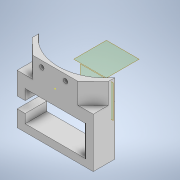
# Autodesk Inventor part: brazo_articulado_2
Saved by Autodesk Inventor 2021 (Build 250183000, 183)
## iProperties
Created: 2021-04-15
Part Number: brazo_articulado_2
Material: Genérico
Document SubType Name: Modeling
Designer: Joaquín
Density: 1 g/cm^3
Appearance: Valor por defecto
Author: Joaquín
Autodesk Inventor part; units mm, degrees
ref_plane "YZ Plane" through (0, 0, 0) normal (1, 0, 0) x (0, 1, 0)
ref_plane "XZ Plane" through (0, 0, 0) normal (0, 1, 0) x (-1, 0, 0)
ref_plane "XY Plane" through (0, 0, 0) normal (0, 0, 1) x (1, 0, 0)
ref_plane "Plano de trabajo1" through (16, 0, 22.5) normal (0, 0, -1) x (-1, 0, 0)
sketch "Boceto2" plane through (16, 0, 22.5) normal (0, 0, -1) x (-1, 0, 0)
  line L0 (-6.5, 0) -> (0, 0) projected
  line L1 (0, 0) -> (32, 0) projected
  circle A0 centre (8, 8) radius 1.5
  circle A1 centre (24, 8) radius 1.5
  point P0 (16, 0)
  dimension "d15" = 3
  dimension "d16" = 3
  constraints: 2 centre point
  measures "d15" diameter of A0
  measures "d16" diameter of A1
extrude "Extrusión2" [suppressed]
ref_plane "Plano de trabajo2" through (0, 0, 0) normal (0, -1, 0) x (1, 0, 0)
sketch "Boceto4" plane through (0, 0, 0) normal (0, -1, 0) x (1, 0, 0)
  circle A0 centre (0, 0) radius 32.5
  arc A1 (28.2887, 16) -> (-28.2887, 16) centre (0, 0) ccw projected
  line L0 (0, 32.5) -> (0, 34.5)
  line L1 (0, 34.5) -> (-26.2329, 34.5)
  line L2 (-26.2329, 34.5) -> (30.7149, 34.5)
  line L3 (0, 0) -> (0, 20)
  arc A2 (28.2887, 16) -> (-28.2887, 16) centre (0, 0) ccw projected
  line L4 (0, 20) -> (50, 20)
  line L5 (50, 20) -> (-50, 20)
  line L6 (0, 34.5) -> (15, 34.5)
  line L7 (15, 34.5) -> (25.6174, 20)
  line L8 (0, 34.5) -> (-15, 34.5)
  line L9 (-15, 34.5) -> (-25.6174, 20)
  point P0 (-25.6174, 20)
  dimension "d19" = 2
  dimension "d20" = 20
  dimension "d21" = 50
  dimension "d22" = 100
  dimension "d23" = 15
  dimension "d24" = 15
  constraints: 20 end point, 6 point on line, 3 point on circle, 2 vertical, 1 centre point, 1 coincident, 1 horizontal, 1 perpendicular
  measures "d19" distance of L0.start L0.end
  measures "d20" distance of L3.start L3.end
  measures "d21" distance of L3.end L4.end
  measures "d22" distance of L4.end L5.end
  measures "d23" distance of L0.end L6.end
  measures "d24" distance of L0.end L8.end
extrude "Extrusión3" add sketch "Boceto4" against normal blind 12 contours A0 L0 L2 L7 | L9 L1 L0 A0
sketch "Boceto5" plane through (-15, 0, 34.5) normal (0, 0, 1) x (1, 0, 0)
  line L0 (30, 0) -> (30, 12) projected
  line L1 (30, 0) -> (30, 8)
  line L2 (30, 8) -> (22, 8)
  line L3 (22, 8) -> (6, 8)
  circle A0 centre (22, 8) radius 1.5
  circle A1 centre (6, 8) radius 1.5
  point P0 (15, 0)
  dimension "d27" = 8
  dimension "d28" = 8
  dimension "d29" = 16
  dimension "d30" = 3
  dimension "d31" = 3
  constraints: 6 end point, 2 centre point, 2 coincident, 2 point on line, 1 perpendicular
  measures "d27" distance of L0.start L1.end
  measures "d28" distance of L1.end L2.end
  measures "d29" distance of L2.end L3.end
  measures "d30" diameter of A0
  measures "d31" diameter of A1
extrude "Extrusión4" cut sketch "Boceto5" against normal blind 12
sketch "Boceto6" plane through (0, 0, 0) normal (0, -1, 0) x (1, 0, 0)
  circle A0 centre (0, 0) radius 32.5
  arc A1 (25.6174, 20) -> (-25.6174, 20) centre (0, 0) ccw projected
  line L0 (-15, 34.5) -> (15, 34.5) projected
  line L1 (25.6174, 20) -> (15, 34.5)
  line L2 (15, 34.5) -> (-15, 34.5)
  line L3 (-15, 34.5) -> (-25.6174, 20)
  constraints: 6 end point, 1 centre point, 1 coincident, 1 collinear, 1 point on circle
extrude "Extrusión5" add sketch "Boceto6" along normal blind 2 contours A0 L3 L0 L1
sketch "Boceto7" plane through (0, -2, 0) normal (0, -1, 0) x (1, 0, 0)
  line L0 (-25.6174, 20) -> (-15, 34.5) projected
  line L1 (-15, 34.5) -> (-25.6174, 34.5)
  line L2 (-25.6174, 34.5) -> (-25.6174, 20)
  line L3 (-25.6174, 20) -> (25.6174, 20)
  line L4 (25.6174, 20) -> (25.6174, 34.5)
  line L5 (25.6174, 20) -> (15, 34.5) projected
  line L6 (15, 34.5) -> (25.6174, 34.5)
  circle A0 centre (0, 0) radius 32.5
  line L7 (-15, 34.5) -> (15, 34.5)
  constraints: 12 end point, 3 horizontal, 3 perpendicular, 1 coincident, 1 point on line, 3 other
extrude "Extrusión6" add sketch "Boceto7" along normal blind 8 contours L2 L1 L0 | A0 L3 | L0 L7 L5 A0 | L5 L6 L4 picked at (-1.7193, 25.9173)
sketch "Boceto8" plane through (-15, 12, 34.5) normal (0, 0, 1) x (1, 0, 0)
  line L0 (40.6174, -22) -> (-10.6174, -22) projected
  line L1 (-10.6174, -22) -> (-10.6174, -42.5)
  line L2 (-10.6174, -42.5) -> (39.7361, -42.5)
  line L3 (40.6174, -22) -> (40.6174, -42.5)
  line L4 (40.6174, -42.5) -> (39.7361, -42.5)
  line L5 (-10.6174, -22) -> (40.6174, -22) projected
  line L6 (40.6174, -14) -> (40.6174, -22) projected
  line L7 (-10.6174, -22) -> (40.6174, -22)
  line L8 (15, -22) -> (35.2, -22)
  line L9 (35.2, -22) -> (35.2, -42.5)
  line L10 (15, -22) -> (-5.2, -22)
  line L11 (-5.2, -22) -> (-5.2, -42.5)
  line L12 (-5.2, -42.5) -> (-5.2, -37.5)
  line L13 (-5.2, -22) -> (-5.2, -29)
  line L14 (-5.2, -29) -> (-10.6174, -29)
  line L15 (-5.2, -42.5) -> (-5.2, -36.5)
  line L16 (-5.2, -36.5) -> (-10.6174, -36.5)
  point P0 (15, -12)
  dimension "d38" = 20.5
  dimension "d39" = 20.5
  dimension "d40" = 20.2
  dimension "d41" = 20.2
  dimension "d43" = 7
  dimension "d44" = 6
  constraints: 28 end point, 9 point on line, 5 perpendicular, 2 vertical, 1 horizontal, 1 midpoint
  measures "d38" distance of L0.end L1.end
  measures "d39" distance of L0.start L3.end
  measures "d40" distance of L8.start L8.end
  measures "d41" distance of L8.start L10.end
  measures "d43" distance of L10.end L13.end
  measures "d44" distance of L11.end L15.end
extrude "Extrusión7" add sketch "Boceto8" against normal blind 14.5 contours L3 L4 L2 L9 L0 | L11 L14 L1 L0 | L2 L1 L16 L11
sketch "Boceto9" plane through (20.2, -30.5, 34.5) normal (0, -1, 0) x (1, 0, 0)
  line L0 (5.4174, -14.5) -> (5.4174, 0) projected
  line L1 (-45.8174, 0) -> (-45.8174, -14.5) projected
  line L2 (5.4174, 0) -> (-45.8174, 0)
  line L3 (-45.8174, 0) -> (-45.8174, -14.5)
  line L4 (-45.8174, -14.5) -> (5.4174, -14.5)
  line L5 (5.4174, 0) -> (-5.2, 0) projected
  line L6 (5.4174, -14.5) -> (5.4174, 0)
  point P0 (-20.2, -34.5)
  constraints: 8 end point, 2 perpendicular, 1 collinear, 1 horizontal
extrude "Extrusión8" add sketch "Boceto9" along normal blind 5
sketch "Boceto10" plane through (0, -2, 0) normal (0, 1, 0) x (1, 0, 0)
  line L0 (-15, -34.5) -> (-25.6174, -34.5) projected
  line L1 (-15, -34.5) -> (-25.6174, -34.5)
  line L2 (-25.6174, -34.5) -> (-25.6174, -24.5)
  line L3 (-25.6174, -34.5) -> (-25.6174, -20) projected
  line L4 (-25.6174, -24.5) -> (-15, -34.5)
  line L5 (-25.6174, -20) -> (25.6174, -20) projected
  line L6 (-25.6174, -24.5) -> (-25.6174, -20)
  line L7 (-25.6174, -20) -> (-15, -34.5)
  line L8 (-15, -34.5) -> (-25.6174, -20) projected
  arc A0 (-25.6174, -20) -> (25.6174, -20) centre (0, 0) ccw projected
  line L9 (0, -32.5) -> (0, -25.3096)
  line L10 (15, -34.5) -> (25.6174, -34.5)
  line L11 (25.6174, -34.5) -> (25.6174, -24.5)
  line L12 (25.6174, -34.5) -> (25.6174, -20)
  line L13 (25.6174, -24.5) -> (15, -34.5)
  line L14 (25.6174, -20) -> (15, -34.5)
  dimension "d49" = 10
  constraints: 22 end point, 5 point on line, 4 symmetric about line, 2 vertical, 1 horizontal, 1 point on circle
  measures "d49" distance of L0.end L2.end
extrude "Extrusión9" add sketch "Boceto10" along normal blind 14 contours L12 L13 L14 | L4 L3 L7
sketch "Boceto11" plane through (-25.6174, -17, 34.5) normal (0, 0, 1) x (1, 0, 0)
  line L0 (45.8174, 7) -> (45.8174, -13.5) projected
  line L1 (45.8174, -13.5) -> (45.8174, 7)
  line L2 (45.8174, 7) -> (45.8174, -3.25)
  point P0 (25.6174, 17)
  constraints: 4 end point, 1 midpoint, 1 vertical
